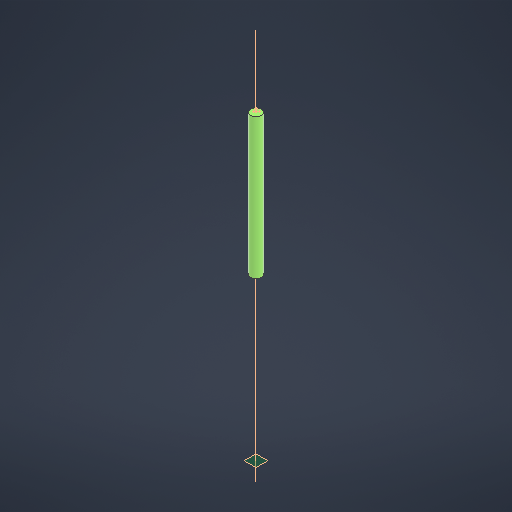
# Autodesk Inventor part: LOOP2_COLL_POSTDEF1
Saved by Autodesk Inventor 2026.1 (Build 301233000, 233)
## iProperties
Created: 2024-08-12
Part Number: LOOP2_COLL_POSTDEF1
Material: Generic
Document SubType Name: Modeling
Designer: User
Density: 1 g/cm^3
Appearance: Default
Author: User
Autodesk Inventor part; units mm, degrees
ref_plane "YZ Plane" through (0, 0, 0) normal (1, 0, 0) x (0, 1, 0)
ref_plane "XZ Plane" through (0, 0, 0) normal (0, 1, 0) x (-1, 0, 0)
ref_plane "XY Plane" through (0, 0, 0) normal (0, 0, 1) x (1, 0, 0)
sketch "Sketch1" plane through (0, 0, 0) normal (0, 1, 0) x (-1, 0, 0)
  circle A0 centre (0, 0) radius 1
  dimension "d0" = 2
  constraints: 1 centre point, 1 coincident
  measures "d0" diameter of A0
extrude "Extrusion1" add sketch "Sketch1" along normal blind 26.057
ref_plane "Work Plane1" through (0, -30, 0) normal (0, -1, 0) x (1, 0, 0)
body "Solid1"
